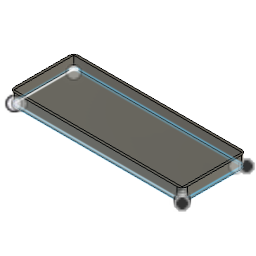
Untitled (Autodesk Fusion 360 design; units mm, degrees)
Autodesk Fusion 360 part; units mm, degrees
sketch "Sketch1" plane through (0, 0, 0) normal (0, 0, 1) x (1, 0, 0)
  line L0 (0, 0) -> (350.815, 0)
  line L1 (350.815, 0) -> (350.815, 124.629)
  line L2 (0, 124.629) -> (0, 0)
  line L3 (350.815, 0) -> (350.815, 124.629)
  line L4 (344.815, 129.629) -> (0, 129.629)
  line L5 (0, 0) -> (0, 124.629)
  line L6 (0, 0) -> (350.815, 0)
  line L7 (0, 129.629) -> (344.815, 129.629)
  line L8 (350.815, 124.629) -> (0, 124.629)
  line L9 (350.815, 124.629) -> (350.815, 0)
  line L10 (355.815, 6) -> (355.815, 118.629)
  line L11 (344.815, -5) -> (6, -5)
  line L12 (-5, -5) -> (-5, 0)
  line L13 (0, 0) -> (350.815, 0)
  line L14 (0, 0) -> (0, 124.629)
  line L15 (0, 129.629) -> (6, 129.629)
  line L16 (-5, 118.629) -> (-5, 6)
  arc A0 (-5, 6) -> (6, -5) centre (6, 6) ccw
  arc A1 (6, 129.629) -> (-5, 118.629) centre (6, 118.629) ccw
  arc A2 (344.815, -5) -> (355.815, 6) centre (344.815, 6) ccw
  arc A3 (355.815, 118.629) -> (344.815, 129.629) centre (344.815, 118.629) ccw
  line L17 (6, 129.629) -> (0, 129.629)
  point P0 (355.815, 129.629)
  point P1 (355.815, -5)
  dimension "d12" = 355.815
  dimension "d13" = 5
  dimension "d16" = 11
  dimension "d17" = 11
  dimension "d18" = 11
  dimension "d19" = 11
  dimension "d24" = 360.815
  dimension "d25" = 134.629
  constraint horizontal L0
  constraint vertical L1
  constraint vertical L2
  constraint coincident L0.start L2.end
  constraint vertical L3
  constraint horizontal L4
  constraint vertical L5
  constraint horizontal L6
  constraint coincident L2 L0.start
  constraint horizontal L7
  constraint horizontal L8
  constraint vertical L9
  constraint vertical L10
  constraint horizontal L11
  constraint vertical L12
  constraint horizontal L13
  constraint vertical L14
  constraint horizontal L15
  constraint vertical L16
  constraint coincident L12.end L16
  constraint coincident L12.start L11
  constraint tangent L16 A0
  constraint tangent L11 A0
  constraint tangent L16 A1
  constraint tangent L15 A1
  constraint coincident P1 L10
  constraint tangent L10 A2
  constraint coincident P0 L7
  constraint tangent L7 A3
  measures "d12" distance of L4.end P0
  measures "d13" distance of L4.end L2.start
  measures "d16" radius of A0
  measures "d17" radius of A1
  measures "d18" radius of A2
  measures "d19" radius of A3
  measures "d24" distance of L10 L16
  measures "d25" distance of L7 L11
extrude "Extrude1" add sketch "Sketch1" along normal blind 3 contours L0 L1 L2 L3 L5 L6 L8 L9 L13 L14
extrude "Extrude2" add sketch "Sketch1" along normal blind 25
equation "d12 = 350.815 mm + 5 mm"
